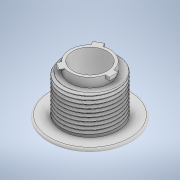
# Autodesk Inventor part: Adapter Male v002
Saved by Autodesk Inventor 2020.2 (Build 242310000, 310)
## iProperties
Created: 2020-04-26
Part Number: Adapter Male v002
Material: Generic
Document SubType Name: Modeling
Designer: a
Density: 1 g/cm^3
Appearance: Default
Author: a
Autodesk Inventor part; units mm, degrees
ref_plane "YZ Plane" through (0, 0, 0) normal (1, 0, 0) x (0, 1, 0)
ref_plane "XZ Plane" through (0, 0, 0) normal (0, 1, 0) x (-1, 0, 0)
ref_plane "XY Plane" through (0, 0, 0) normal (0, 0, 1) x (1, 0, 0)
sketch "Sketch1" plane through (0, 0, 0) normal (0, 1, 0) x (-1, 0, 0)
  circle A0 centre (0, 0) radius 22.5
  dimension "d0" = 45
  constraints: 1 centre point, 1 coincident
  measures "d0" diameter of A0
extrude "Extrusion1" add sketch "Sketch1" along normal blind 2
fillet "Fillet1" radius 1 2 edges at (22.5, 2, 0) (22.5, 0, 0)
sketch "Sketch2" plane through (0, 2, 0) normal (0, 1, 0) x (1, 0, 0)
  circle A0 centre (0, 0) radius 15
  dimension "d3" = 30
  constraints: 1 centre point, 1 coincident
  measures "d3" diameter of A0
extrude "Thread_L" add sketch "Sketch2" along normal blind 20
sketch "Sketch3" plane through (0, 22, 0) normal (0, 1, 0) x (1, 0, 0)
  circle A0 centre (0, 0) radius 10.75
  dimension "d7" = 21.5
  constraints: 1 centre point, 1 coincident
  measures "d7" diameter of A0
extrude "Tube_L" add sketch "Sketch3" along normal blind 5
sketch "Sketch4" plane through (0, -2.12, 0) normal (1, 0, 0) x (0, 1, 0)
  line L0 (29.12, 0) -> (29.12, 2.35)
  line L1 (29.12, 2.35) -> (27.47, 2.35)
  line L2 (27.47, 2.35) -> (27.47, -0.85)
  line L3 (29.12, 0) -> (29.12, -2.35)
  line L4 (29.12, -2.35) -> (28.97, -2.35)
  line L5 (28.97, -2.35) -> (27.47, -0.85)
  line L6 (-2.9407, 0) -> (32.4843, 0) projected
  line L7 (29.12, -10.75) -> (29.12, 10.75) projected
  dimension "d14" = 2.35
  dimension "d13" = 1.65
  dimension "d12" = 3.2
  dimension "d11" = 2.35
  dimension "d10" = 0.15
  constraints: 12 end point, 2 perpendicular, 2 vertical, 1 horizontal, 1 midpoint, 1 point on line
  measures "d14" distance of L0.start L0.end
  measures "d13" distance of L0.end L1.end
  measures "d12" distance of L1.end L2.end
  measures "d11" distance of L0.start L3.end
  measures "d10" distance of L3.end L4.end
extrude "Bayonet Tab" add sketch "Sketch4" along normal blind 12.75 separate body
pattern_circular "Circular Pattern1" count 3 over 360 about axis through (0, -10, 0) along (0, 1, 0) of "Bayonet Tab"
sketch "Sketch5" plane through (0, 0, 0) normal (0, -1, 0) x (1, 0, 0)
  circle A0 centre (0, 0) radius 9.25
  dimension "d21" = 18.5
  constraints: 1 centre point, 1 coincident
  measures "d21" diameter of A0
extrude "Extrusion5" cut sketch "Sketch5" against normal through all
thread "Thread4" size "M30x2" class "6g" standard "ANSI Metric M Profile" full length
sketch "Sketch15" plane through (0, 22, 0) normal (-1, 0, 0) x (0, -1, 0)
  line L0 (-1.1668, -13.6184) -> (-1.0001, -13.6184) construction
  line L1 (0.1666, -14.899) -> (-0.0001, -15.2192) construction
  line L2 (-2.0001, -15.2192) -> (-2.1668, -14.899) construction
  line L3 (-0.8334, -13.6184) -> (-1.0001, -13.2982) construction
  line L4 (-1.0001, -13.2982) -> (-1.1668, -13.6184) construction
  line L5 (-2.0001, -15.2192) -> (-1.8334, -14.899) construction
  line L6 (-0.8334, -13.6184) -> (-0.1668, -14.899)
  line L7 (-2.1668, -14.899) -> (-1.8334, -14.899) construction
  arc A0 (-2.1668, -14.899) -> (-2.0001, -15.0002) centre (-2.0001, -14.8123) ccw construction
  line L8 (0.1666, -14.899) -> (-0.1668, -14.899) construction
  line L9 (-2.0001, -15.2192) -> (-2.0001, -14.899) construction
  line L10 (-0.0001, -15.2192) -> (-0.0001, -14.899) construction
  line L11 (-1.0001, -13.2982) -> (-1.0001, -13.5172) construction
  line L12 (-2.0001, -15.0002) -> (-0.0001, -15.0002)
  arc A1 (-2.0001, -15.0002) -> (-1.8334, -14.899) centre (-2.0001, -14.8123) ccw
  line L13 (-0.1668, -14.899) -> (-0.0001, -15.2192) construction
  line L14 (-1.8334, -14.899) -> (-1.1668, -13.6184)
  line L15 (-0.0001, -0.0002) -> (-0.0001, 0.0177)
  line L16 (-0.0001, 0.0177) -> (-0.0001, -0.0002)
  line L17 (-0.0001, -0.0002) -> (0.0334, -0.0002)
  arc A2 (-0.1668, -14.899) -> (-0.0001, -15.0002) centre (-0.0001, -14.8123) ccw
  arc A3 (-0.0001, -15.0002) -> (0.1666, -14.899) centre (-0.0001, -14.8123) ccw construction
  arc A4 (-1.0001, -13.5172) -> (-1.1668, -13.6184) centre (-1.0001, -13.7051) ccw
  arc A5 (-0.8334, -13.6184) -> (-1.0001, -13.5172) centre (-1.0001, -13.7051) ccw
  line L18 (-1.0001, -13.5172) -> (-1.0001, -13.6184) construction
  line L19 (-1.0001, -13.6184) -> (-0.8334, -13.6184) construction
  dimension "d89" = 55
  dimension "d90" = 0.3202
  dimension "d91" = 0.3202
  dimension "Sketch15_ThreadOffset" = 0
  dimension "Sketch15_MajorRadius" = 15
  dimension "d94" = 2
  dimension "Sketch15_MinorRadius" = 13.5171
  constraints: 40 end point, 12 point on circle, 10 parallel, 8 tangent, 6 centre point, 6 collinear, 2 midpoint, 2 point on line, 1 horizontal, 1 perpendicular, 3 other
  measures "d89" angle of L6 L14
  measures "d90" distance of L3.end L0.end
  measures "d91" distance of L1.end L10.end
  measures "Sketch15_ThreadOffset" distance between parallel lines of L15 L10
  measures "Sketch15_MajorRadius" distance from line of L12 L15.start
  measures "d94" distance from line of L1.end L9
  measures "Sketch15_MinorRadius" distance edge to line of A5 L17
sketch "Sketch16" plane through (0, 22, 0) normal (1, 0, 0) x (0, 0, 1)
  line L0 (15, 0) -> (15, 20)
  line L1 (15, 20) -> (13.5171, 20)
  line L2 (13.5171, 20) -> (13.5171, 0)
  line L3 (13.5171, 0) -> (15, 0)
  line L4 (0, -10.4) -> (0, 27.4) projected
  constraints: 8 end point
revolve "Revolution7" [suppressed]
sketch "Sketch17" plane through (0, 22, 0) normal (1, 0, 0) x (0, 0, 1)
  line L0 (15, 0) -> (15, 20)
  line L1 (15, 20) -> (13.5171, 20)
  line L2 (13.5171, 20) -> (13.5171, 0)
  line L3 (13.5171, 0) -> (15, 0)
  line L4 (0, -10.4) -> (0, 27.4) projected
  constraints: 8 end point
revolve "Revolution8" [suppressed]
coil "Coil4" sketch "Sketch15" operation cut axis through (0, 22, 0) along (0, -1, 0) pitch 2.002 turns 9.99001 hand right
equation "\"d0\" = Washer_D"
equation "\"d1\" = Washer_T"
equation "\"d6\" = 0.5 * Washer_T"
equation "\"d3\" = Thread_D"
equation "\"d4\" = Thread_L"
equation "\"d7\" = Tube_D"
equation "\"d8\" = Tube_L"
equation "\"d21\" = Hole_D"
equation "\"d89\" = d96"
equation "\"d90\" = 0.160083 * Sketch15_Pitch"
equation "\"d91\" = 0.160083 * Sketch15_Pitch"
equation "\"d94\" = Sketch15_Pitch"
equation "\"Thread_D\" = 30"
equation "\"Washer_D\" = 45"
equation "\"Washer_T\" = 2"
equation "\"Thread_L\" = 20"
equation "\"Tube_D\" = 21.5"
equation "\"Tube_L\" = 5"
equation "\"Hole_D\" = 18.5"
equation "\"d33\" = 55deg"
equation "\"Sketch6_Pitch\" = 1"
equation "\"d54\" = 55deg"
equation "\"Sketch9_Pitch\" = 1"
equation "\"d75\" = 55deg"
equation "\"Sketch12_Pitch\" = 1"
equation "\"d96\" = 55deg"
equation "\"Sketch15_Pitch\" = 2"
body "Solid1"
body "Solid5"
